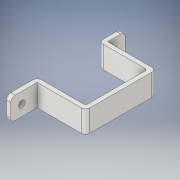
# Autodesk Inventor part: Akkuhalterung
Saved by Autodesk Inventor 2018 (Build 220112000, 112)
## iProperties
Created: 2019-03-04
Part Number: Akkuhalterung
Material: ABS-Kunststoff
Document SubType Name: Modeling
Designer: RedBots
Density: 1.06 g/cm^3
Appearance: Glatt - weiß
Mass: 1.9661 g
Surface Area: 22.9076 cm^2
Volume: 1.85481 cm^3
Author: RedBots
Autodesk Inventor part; units mm, degrees
ref_plane "YZ Plane" through (0, 0, 0) normal (1, 0, 0) x (0, 1, 0)
ref_plane "XZ Plane" through (0, 0, 0) normal (0, 1, 0) x (-1, 0, 0)
ref_plane "XY Plane" through (0, 0, 0) normal (0, 0, 1) x (1, 0, 0)
sketch "Skizze1" plane through (0, 0, 0) normal (0, 0, 1) x (1, 0, 0)
  line L0 (0, 0) -> (22, 0)
  line L1 (22, 0) -> (22, 28)
  line L2 (22, 28) -> (0, 28)
  line L3 (0, 28) -> (0, 38)
  line L4 (0, 38) -> (2, 38)
  line L5 (2, 38) -> (2, 30)
  line L6 (2, 30) -> (24, 30)
  line L7 (24, 30) -> (24, -2)
  line L8 (24, -2) -> (2, -2)
  line L9 (2, -2) -> (2, -14)
  line L10 (2, -14) -> (0, -14)
  line L11 (0, -14) -> (0, 0)
  line L12 (22, 0) -> (22, -2) construction
  line L13 (22, 28) -> (22, 30) construction
  dimension "d1" = 14
  dimension "d3" = 2
  dimension "d4" = 20
  dimension "d5" = 2
  dimension "d6" = 28
  dimension "d7" = 2
  dimension "d17" = 10
  constraints: 28 end point, 10 perpendicular, 3 equal length, 3 point on line, 2 horizontal, 1 vertical
  measures "d1" distance of L10.end L0.start
  measures "d3" distance between parallel lines of L8 L0
  measures "d4" distance between parallel lines of L1 L5
  measures "d5" distance between parallel lines of L7 L1
  measures "d6" distance between parallel lines of L0 L2
  measures "d7" distance between parallel lines of L9 L11
  measures "d17" distance of L2.end L3.end
extrude "Extrusion1" add sketch "Skizze1" along normal blind 10
fillet "Rundung1" radius 2 4 edges at (0, 28, 5) (0, 0, 5) (24, 30, 5) (24, -2, 5)
fillet "Rundung2" radius 2 4 edges at (1, -14, 10) (1, -14, 0) (1, 38, 10) (1, 38, 0)
sketch "Skizze2" plane through (0, 30, 0) normal (-1, 0, 0) x (0, 0, 1)
  line L0 (2, 8) -> (8, 8) construction
  line L1 (5, 8) -> (5, -2) construction
  line L2 (0, -2) -> (10, -2) construction
  circle A0 centre (5, 3) radius 1.5
  line L3 (10, -2) -> (10, -30) construction
  line L4 (0, -2) -> (0, -30) construction
  circle A1 centre (5, -39) radius 1.5
  line L5 (0, -32) -> (10, -32) projected
  point P0 (10, -4)
  point P1 (10, -28)
  point P2 (0, -4)
  point P3 (0, -28)
  point P4 (0, 0)
  dimension "d12" = 3
  dimension "d15" = 3
  dimension "d18" = 7
  constraints: 3 midpoint, 2 centre point, 2 end point
  measures "d12" diameter of A0
  measures "d15" vertical distance of point (0, 0) A0.centre
  measures "d18" distance from line of L5 A1.centre
extrude "Extrusion2" cut sketch "Skizze2" against normal up to next
fillet "Rundung3" radius 1 2 edges at (22, 28, 5) (22, 0, 5)
